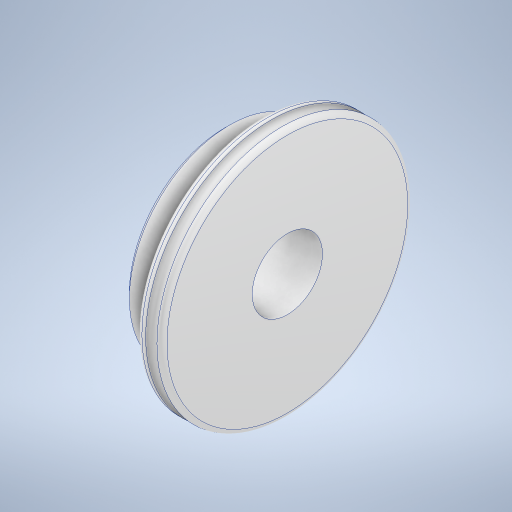
# Autodesk Inventor part: IDLE ROLLER END CAP
Saved by Autodesk Inventor 2023 (Build 270158000, 158)
## iProperties
Created: 2022-08-21
Part Number: IDLE ROLLER END CAP
Material: Aluminum 6061
Document SubType Name: Modeling
Designer: D.C. Eksteen
Density: 2.7 g/cm^3
Appearance: Aluminum - Flat
Mass: 374.408 g
Surface Area: 235.525 cm^2
Volume: 138.67 cm^3
Author: D.C. Eksteen
Title: FRONT ROLLER END CAP
Autodesk Inventor part; units mm, degrees
ref_plane "YZ Plane" through (0, 0, 0) normal (1, 0, 0) x (0, 1, 0)
ref_plane "XZ Plane" through (0, 0, 0) normal (0, 1, 0) x (-1, 0, 0)
ref_plane "XY Plane" through (0, 0, 0) normal (0, 0, 1) x (1, 0, 0)
sketch "Sketch1" plane through (0, 0, 0) normal (0, 0, 1) x (1, 0, 0)
  line L0 (0, 0) -> (25, 0)
  line L1 (25, 0) -> (25, 50)
  line L2 (15, 50) -> (15, 40)
  line L3 (15, 40) -> (0, 40)
  line L4 (0, 40) -> (0, 0)
  line L5 (15, 50) -> (18.5, 50)
  line L6 (18.5, 50) -> (18.5, 47)
  line L7 (18.5, 47) -> (23, 47) construction
  line L8 (23, 47) -> (23, 50)
  line L9 (23, 50) -> (25, 50)
  circle A0 centre (20.75, 50) radius 2.25 construction
  line L10 (18.5, 50) -> (23, 50) construction
  arc A1 (18.5, 50) -> (23, 50) centre (20.75, 50) ccw
  point P0 (23, 48.5)
  point P1 (20.75, 50)
  dimension "d1" = 40
  dimension "d2" = 15
  dimension "d3" = 10
  dimension "d5" = 50
  dimension "d6" = 3
  dimension "d7" = 4.5
  dimension "d8" = 2
  constraints: 22 end point, 7 perpendicular, 3 horizontal, 3 midpoint, 2 point on circle, 2 tangent, 1 centre point, 1 horizontal alignment, 1 point on line, 1 vertical, 2 other
  measures "d1" distance between parallel lines of L0 L3
  measures "d2" distance between parallel lines of L4 L2
  measures "d3" distance between parallel lines of L1 L2
  measures "d5" distance from line of L0 L1.end
  measures "d6" distance between parallel lines of L9 L7
  measures "d7" distance of L6.end L7.end
  measures "d8" distance from line of L1 point (23, 48.5)
revolve "Revolution1" add sketch "Sketch1" angle 360 about axis through (0, 0, 0) along (1, 0, 0)
fillet "Fillet2" radius 2 1 edges at (15, -50, 0)
fillet "Fillet3" radius 2 1 edges at (25, -50, 0)
chamfer "Chamfer1" distance 2 angle 45 1 edges at (0, -40, 0)
sketch "Sketch2" plane through (25, 0, 0) normal (1, 0, 0) x (0, 0, -1)
  circle A0 centre (0, 0) radius 48 projected
  constraints: 1 coincident
hole "Hole1" at (25, 0, 0) direction (-1, 0, 0) diameter 20 end through all
sketch "Sketch3" plane through (25, 0, 0) normal (1, 0, 0) x (0, 0, -1)
  circle A0 centre (0, 0) radius 10 projected
  circle A1 centre (0, 0) radius 48 projected
  constraints: 1 coincident
hole "Hole2" at (25, 0, 0) direction (-1, 0, 0) diameter 28 depth 22
body "Solid1"
